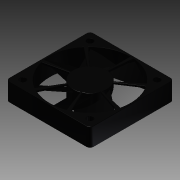
# Autodesk Inventor part: CoolingFan50x50-V01
Saved by Autodesk Inventor 2015 (Build 190159000, 159)
## iProperties
Created: 2014-04-26
Part Number: CoolingFan50x50-V01
Material: Generic
Document SubType Name: Modeling
Designer: spichelh
Density: 1 g/cm^3
Appearance: Default
Author: spichelh
Autodesk Inventor part; units mm, degrees
ref_plane "YZ Plane" through (0, 0, 0) normal (1, 0, 0) x (0, 1, 0)
ref_plane "XZ Plane" through (0, 0, 0) normal (0, 1, 0) x (-1, 0, 0)
sketch "Sketch2" plane through (0, 0, 0) normal (0, 1, 0) x (-1, 0, 0)
  line L0 (2, 0) -> (48, 0)
  line L1 (50, -2) -> (50, -48)
  line L2 (48, -50) -> (2, -50)
  line L3 (0, -48) -> (0, -2)
  circle A0 centre (5, -45) radius 1.75
  line L4 (0, -25) -> (7.2636, -25) construction
  line L5 (25, -50) -> (25, -40.7459) construction
  circle A1 centre (5, -5) radius 1.75
  circle A2 centre (45, -45) radius 1.75
  circle A3 centre (45, -5) radius 1.75
  arc A4 (2, 0) -> (0, -2) centre (2, -2) ccw
  arc A5 (0, -48) -> (2, -50) centre (2, -48) ccw
  arc A6 (48, -50) -> (50, -48) centre (48, -48) ccw
  arc A7 (50, -2) -> (48, 0) centre (48, -2) ccw
  circle A8 centre (25, -25) radius 24
  circle A9 centre (25, -25) radius 10
  point P0 (0, 0)
  point P1 (50, -50)
  point P2 (50, 0)
  point P3 (0, -50)
  dimension "d4" = 50
  dimension "d5" = 50
  dimension "d6" = 40
  dimension "d7" = 40
  dimension "d8" = 3.5
  dimension "d9" = 2
  dimension "d10" = 2
  dimension "d11" = 48
  dimension "d14" = 2
  dimension "d15" = 2
  dimension "d16" = 20
  constraints: 12 end point, 10 centre point, 10 point on line, 8 point on circle, 8 tangent, 3 perpendicular, 3 symmetric about line, 2 equal radius, 2 midpoint, 2 parallel, 1 coincident, 1 horizontal, 3 other
  measures "d4" distance of point (50, -50) point (0, -50)
  measures "d5" distance of point (50, 0) point (50, -50)
  measures "d6" distance of A1.centre A0.centre
  measures "d7" distance of A3.centre A1.centre
  measures "d8" diameter of A0
  measures "d9" radius of A4
  measures "d10" radius of A5
  measures "d11" diameter of A8
  measures "d14" radius of A7
  measures "d15" radius of A6
  measures "d16" diameter of A9
extrude "Extrusion2" add sketch "Sketch2" along normal blind 10.7
sketch "Sketch3" plane through (0, 10.7, 0) normal (0, 1, 0) x (1, 0, 0)
  circle A0 centre (-25, 25) radius 24 projected
  line L0 (-2, 50) -> (-48, 50) projected
  line L1 (-25, 25) -> (-25, 50)
  line L2 (-25, 25) -> (-22.8211, 49.9049)
  arc A1 (-22.8211, 49.9049) -> (-25, 50) centre (-25, 25) ccw
  line L3 (-25, 25) -> (-44.5458, 40.5872)
  line L4 (-25, 25) -> (-43.1129, 42.2315)
  arc A2 (-43.1129, 42.2315) -> (-44.5458, 40.5872) centre (-25, 25) ccw
  line L5 (-25, 25) -> (-49.3732, 19.437)
  line L6 (-25, 25) -> (-49.7653, 21.5824)
  arc A3 (-49.7653, 21.5824) -> (-49.3732, 19.437) centre (-25, 25) ccw
  line L7 (-25, 25) -> (-35.8471, 2.4758)
  line L8 (-25, 25) -> (-37.7689, 3.5069)
  arc A4 (-37.7689, 3.5069) -> (-35.8471, 2.4758) centre (-25, 25) ccw
  line L9 (-25, 25) -> (-14.1529, 2.4758)
  line L10 (-25, 25) -> (-16.1573, 1.6161)
  arc A5 (-16.1573, 1.6161) -> (-14.1529, 2.4758) centre (-25, 25) ccw
  line L11 (-25, 25) -> (-0.6268, 19.437)
  line L12 (-25, 25) -> (-1.2044, 17.3339)
  arc A6 (-1.2044, 17.3339) -> (-0.6268, 19.437) centre (-25, 25) ccw
  line L13 (-25, 25) -> (-5.4542, 40.5872)
  line L14 (-25, 25) -> (-4.1701, 38.8244)
  arc A7 (-4.1701, 38.8244) -> (-5.4542, 40.5872) centre (-25, 25) ccw
  point P0 (0, 0)
  dimension "d25" = 5
  dimension "d32" = 360
  constraints: 28 end point, 14 point on circle, 7 centre point, 2 coincident, 1 midpoint, 41 other
  measures "d25" angle of L1 L2
extrude "Extrusion3" add sketch "Sketch3" against normal blind 1 contours L14 L13 A0 | A0 L13 A7 L14 | L11 A6 L12 A0 | A0 L12 L11 | L1 A0 L2 | L3 A0 L4 | L5 A0 L6 | L7 A0 L8 | L9 A0 L10 | A0 L1 A1 L2 | L3 A2 L4 A0 | L5 A3 L6 A0 | L7 A4 L8 A0 | L9 A5 L10 A0
sketch "Sketch4" plane through (0, 10.7, 0) normal (0, 1, 0) x (1, 0, 0)
  arc A0 (-48.3983, 19.6595) -> (-37.2582, 4.3666) centre (-25, 25) ccw projected
  line L0 (-34.7493, 22.7748) -> (-48.3983, 19.6595) projected
  arc A1 (-34.7493, 22.7748) -> (-30.1076, 16.4028) centre (-25, 25) ccw projected
  line L1 (-37.2582, 4.3666) -> (-30.1076, 16.4028) projected
  arc A2 (-6.236, 39.9638) -> (-22.9083, 48.9087) centre (-25, 25) ccw projected
  line L2 (-17.1817, 31.2349) -> (-6.236, 39.9638) projected
  arc A3 (-17.1817, 31.2349) -> (-24.1284, 34.9619) centre (-25, 25) ccw projected
  line L3 (-22.9083, 48.9087) -> (-24.1284, 34.9619) projected
  arc A4 (-43.764, 39.9638) -> (-48.7747, 21.7191) centre (-25, 25) ccw projected
  line L4 (-32.8183, 31.2349) -> (-43.764, 39.9638) projected
  arc A5 (-32.8183, 31.2349) -> (-34.9061, 23.633) centre (-25, 25) ccw projected
  line L5 (-48.7747, 21.7191) -> (-34.9061, 23.633) projected
  line L6 (-29.3388, 15.9903) -> (-35.4132, 3.3767) projected
  arc A6 (-29.3388, 15.9903) -> (-21.4629, 15.6464) centre (-25, 25) ccw projected
  line L7 (-16.511, 2.5515) -> (-21.4629, 15.6464) projected
  arc A7 (-35.4132, 3.3767) -> (-16.511, 2.5515) centre (-25, 25) ccw projected
  line L8 (-20.6612, 15.9903) -> (-14.5868, 3.3767) projected
  arc A8 (-20.6612, 15.9903) -> (-15.4818, 21.9336) centre (-25, 25) ccw projected
  line L9 (-2.1562, 17.6405) -> (-15.4818, 21.9336) projected
  arc A9 (-14.5868, 3.3767) -> (-2.1562, 17.6405) centre (-25, 25) ccw projected
  line L10 (-15.2507, 22.7748) -> (-1.6017, 19.6595) projected
  arc A10 (-15.2507, 22.7748) -> (-16.668, 30.5298) centre (-25, 25) ccw projected
  line L11 (-5.0033, 38.2714) -> (-16.668, 30.5298) projected
  arc A11 (-1.6017, 19.6595) -> (-5.0033, 38.2714) centre (-25, 25) ccw projected
  line L12 (-25, 35) -> (-25, 49) projected
  arc A12 (-25, 35) -> (-32.2452, 31.8926) centre (-25, 25) ccw projected
  line L13 (-42.3884, 41.5422) -> (-32.2452, 31.8926) projected
  arc A13 (-25, 49) -> (-42.3884, 41.5422) centre (-25, 25) ccw projected
  line L14 (-2, 50) -> (-48, 50) projected
  arc A14 (-48, 50) -> (-50, 48) centre (-48, 48) ccw projected
  line L15 (-50, 48) -> (-50, 2) projected
  arc A15 (-50, 2) -> (-48, 0) centre (-48, 2) ccw projected
  line L16 (-48, 0) -> (-2, 0) projected
  arc A16 (-2, 0) -> (0, 2) centre (-2, 2) ccw projected
  line L17 (0, 2) -> (0, 48) projected
  arc A17 (0, 48) -> (-2, 50) centre (-2, 48) ccw projected
  circle A18 centre (-45, 45) radius 1.75 projected
  circle A19 centre (-45, 5) radius 1.75 projected
  circle A20 centre (-5, 5) radius 1.75 projected
  circle A21 centre (-5, 45) radius 1.75 projected
  point P0 (0, 0)
  constraints: 1 coincident
ref_plane "Work Plane1" through (-25, 10.7, -25) normal (0, 0, 1) x (1, 0, 0)
sketch "Sketch5" plane through (-25, 10.7, -25) normal (0, 0, 1) x (1, 0, 0)
  line L0 (3.5371, -1) -> (3.5371, 0) construction
  line L1 (-4.3388, 0) -> (3.5371, 0) construction
  line L2 (-4.3388, 0) -> (-4.3388, -1) construction
  line L3 (-4.3388, -1) -> (-5.1076, -1) construction
  line L4 (-5.1076, -1) -> (-5.1076, 0) construction
  line L5 (-9.7493, 0) -> (-5.1076, 0) construction
  line L6 (-9.7493, 0) -> (-9.7493, -1) construction
  line L7 (-9.7493, -1) -> (-9.9061, -1) construction
  line L8 (-9.9061, -1) -> (-9.9061, 0) construction
  line L9 (-7.8183, 0) -> (-9.9061, 0) construction
  line L10 (-7.8183, 0) -> (-7.8183, -1) construction
  line L11 (-7.8183, -1) -> (-7.2452, -1) construction
  line L12 (-7.2452, -1) -> (-7.2452, 0) construction
  line L13 (0, 0) -> (-7.2452, 0) construction
  line L14 (0, 0) -> (0, -1) construction
  line L15 (0, -1) -> (0.8716, -1) construction
  line L16 (0.8716, -1) -> (0.8716, 0) construction
  line L17 (7.8183, 0) -> (0.8716, 0) construction
  line L18 (7.8183, 0) -> (7.8183, -1) construction
  line L19 (7.8183, -1) -> (8.332, -1) construction
  line L20 (8.332, -1) -> (8.332, 0) construction
  line L21 (9.7493, 0) -> (8.332, 0) construction
  line L22 (9.7493, 0) -> (9.7493, -1) construction
  line L23 (9.7493, -1) -> (9.5182, -1) construction
  line L24 (9.5182, -1) -> (9.5182, 0) construction
  line L25 (4.3388, 0) -> (9.5182, 0) construction
  line L26 (4.3388, 0) -> (4.3388, -1) construction
  line L27 (4.3388, -1) -> (3.5371, -1) construction
  line L28 (-10, -10.7) -> (10, -10.7) construction
  line L29 (0, 0) -> (0, -4.5871) construction
  line L30 (-7.7076, -10.1) -> (7.7076, -1.2)
  line L31 (7.7076, -1.2) -> (7.9386, -1.6)
  line L32 (7.9386, -1.6) -> (-7.4767, -10.5)
  line L33 (-7.4767, -10.5) -> (-7.7076, -10.1)
  line L34 (-10, -10.7) -> (-10, 0) construction
  point P0 (25, -10.7)
  point P1 (0, -5.65)
  dimension "d37" = 60
  dimension "d38" = 0.4
  dimension "d41" = 0.2
  dimension "d45" = 0.2
  constraints: 10 end point, 3 perpendicular, 1 midpoint, 1 parallel, 1 point on line
  measures "d37" angle of L29 L30
  measures "d38" vertical distance of L30.start L32.end
  measures "d41" distance from line of L28 L32.end
  measures "d45" distance from line of L27 L30.end
extrude "Extrusion4" add sketch "Sketch5" along normal blind 23.8
sketch "Sketch6" plane through (-25, 10.7, -25) normal (0, 0, 1) x (1, 0, 0)
  line L0 (0, 0) -> (0, 6.8998)
  point P0 (25, -10.7)
  dimension "d46" = 6.8998
  constraints: 2 end point, 1 coincident, 1 vertical
  measures "d46" distance of L0.start L0.end
pattern_circular "Circular Pattern1" count 7 over 360 about axis through (-25, 0, -25) along (0, 1, 0) of "Extrusion4"
fillet "Fillet1" radius 0.2 43 edges at (-0.5858, 10.7, -0.5858) (0, 10.7, -25) (-0.5858, 10.7, -49.4142) (-13.5, 10.7, -50) (-36.5, 10.7, -50) (-49.4142, 10.7, -49.4142) (-50, 10.7, -25) (-49.4142, 10.7, -0.5858) (-25, 10.7, 0) (-17.4611, 10.7, -18.43) (-17.624, 10.7, -9.6835) (-6.9066, 10.7, -9.232) (-8.819, 10.7, -19.787) (-8.4262, 10.7, -21.2171) (-1.3911, 10.7, -29.3148) (-10.8356, 10.7, -34.4006) (-11.7089, 10.7, -35.5993) (-13.6535, 10.7, -46.1485) (-3.25, 10.7, -45) (-3.25, 10.7, -5) (-43.25, 10.7, -5) (-41.5738, 10.7, -21.2171) (-44.3988, 10.7, -10.869) (-43.25, 10.7, -45) (-34.4388, 10.7, -28.3028) (-34.9765, 10.7, -24.3149) (-38.2911, 10.7, -35.5993) (-37.3168, 10.7, -36.7174) (-28.9417, 10.7, -34.1904) (-25, 10.7, -42) (-23.5184, 10.7, -41.9353) (-20.2723, 10.7, -33.8119) (-25.4362, 10.7, -15.0095) (-32.376, 10.7, -9.6835) (-33.0828, 10.7, -19.1121) (-33.6829, 10.7, -10.3847) (-26.0469, 10.7, -1.0228) (-18.987, 10.7, -9.099) (-15.1629, 10.7, -26.7978) (-41.8404, 10.7, -22.676) (-47.6532, 10.7, -32.9267) (-48.9436, 10.7, -23.3557) (-34.4601, 10.7, -47.0569)
body "Solid1"
